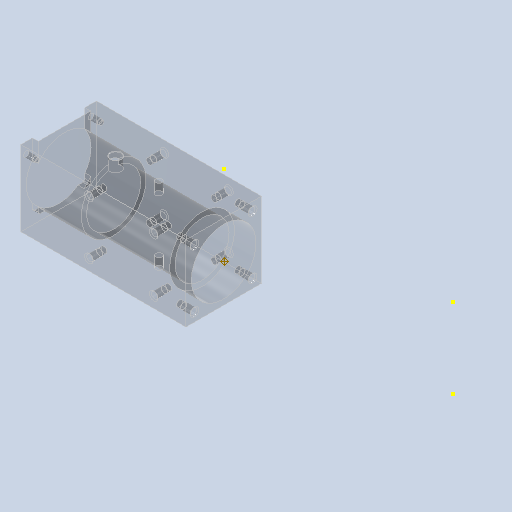
# Autodesk Inventor part: АНЦП.014.00.00.003
Saved by Autodesk Inventor 2022 (Build 260153000, 153)
## iProperties
Created: 2022-02-10
Part Number: АНЦП.014.00.00.003
Material: PET Plastic
Document SubType Name: Modeling
Designer: br4ch
Density: 1.541 g/cm^3
Appearance: Polycarbonate - Clear
Mass: 72.9835 g
Surface Area: 195.713 cm^2
Volume: 47.3611 cm^3
Author: br4ch
Autodesk Inventor part; units mm, degrees
sketch "Sketch1" plane through (0, 0, 0) normal (0, 0, 1) x (1, 0, 0)
  line L0 (-183, -19.5) -> (-106.5, -19.5)
  line L1 (-106.5, -19.5) -> (-106.5, -54.5)
  line L2 (-106.5, -54.5) -> (-183, -54.5)
  line L3 (-183, -54.5) -> (-183, -19.5)
  line L4 (-194, -37) -> (-96, -37) construction
  line L5 (-183, -22) -> (-157.5, -22)
  line L6 (-157.5, -22) -> (-157.5, -37)
  line L7 (-157.5, -24.5) -> (-116.5, -24.5)
  line L8 (-116.5, -37) -> (-116.5, -22)
  line L9 (-116.5, -22) -> (-106.5, -22)
  line L10 (-183, -52) -> (-157.5, -52) construction
  line L11 (-157.5, -52) -> (-157.5, -37) construction
  line L12 (-157.5, -49.5) -> (-116.5, -49.5) construction
  line L13 (-116.5, -37) -> (-116.5, -52) construction
  line L14 (-116.5, -52) -> (-106.5, -52) construction
  line L15 (-183, -37) -> (-106.5, -37)
  point P0 (0, 0)
  dimension "d0" = 76.5
  dimension "d1" = 35
  dimension "d2" = 30
  dimension "d3" = 25.5
  dimension "d4" = 10
  dimension "d5" = 25
  dimension "d6" = 30
  constraints: 32 end point, 9 point on line, 6 symmetric about line, 5 perpendicular, 3 horizontal, 2 midpoint, 2 parallel
  measures "d0" distance of L1.end L2.end
  measures "d1" distance of L0.end L1.end
  measures "d2" distance between parallel lines of L10 L5
  measures "d3" distance of L10.start L10.end
  measures "d4" distance of L13.end L14.end
  measures "d5" distance between parallel lines of L12 L7
  measures "d6" distance between parallel lines of L14 L9
sketch "Sketch3" plane through (0, 0, 0) normal (1, 0, 0) x (0, 1, 0)
  point P0 (0, 0)
ref_plane "Work Plane1" through (-106.5, -37, 0) normal (1, 0, 0) x (0, 1, 0)
sketch "Sketch4" plane through (-106.5, -37, 0) normal (1, 0, 0) x (0, 1, 0)
  point P0 (37, 0)
sketch "Sketch5" plane through (-106.5, -37, 0) normal (1, 0, 0) x (0, 1, 0)
  line L0 (-17.5, 17.5) -> (17.5, 17.5)
  line L1 (17.5, 17.5) -> (17.5, -17.5)
  line L2 (17.5, -17.5) -> (-17.5, -17.5)
  line L3 (-17.5, -17.5) -> (-17.5, 17.5)
  line L4 (-17.5, 17.5) -> (17.5, -17.5) construction
  line L5 (17.5, 17.5) -> (-17.5, -17.5) construction
  point P0 (37, 0)
  point P1 (0, 0)
  dimension "d10" = 35
  dimension "d11" = 35
  constraints: 12 end point, 2 midpoint, 2 parallel, 1 horizontal, 1 perpendicular
  measures "d10" distance of L1.end L2.end
  measures "d11" distance of L0.end L1.end
ref_plane "Work Plane2" through (-183, -37, 0) normal (1, 0, 0) x (0, 1, 0)
extrude "Extrusion1" add sketch "Sketch5" against normal up to surface (76.5 mm away)
revolve "Revolution2" cut sketch "Sketch1" angle 360 about axis through (-194, -37, 0) along (1, 0, 0) contours L5 L6 L15 L3 | L1 L15 L8 L9 | L6 L7 L8 L15
sketch "Sketch7" plane through (-106.5, -37, 0) normal (1, 0, 0) x (0, 0, -1)
  circle A0 centre (0, 0) radius 19.09
  line L0 (-17.5, -17.5) -> (17.5, -17.5) projected
  line L1 (-17.5, 17.5) -> (-17.5, -17.5) projected
  line L2 (17.5, -17.5) -> (-17.5, 17.5) construction
  circle A1 centre (13.4987, -13.4987) radius 1.5
  circle A2 centre (13.4987, 13.4987) radius 1.5
  circle A3 centre (-13.4987, 13.4987) radius 1.5
  circle A4 centre (-13.4987, -13.4987) radius 1.5
  point P0 (0, 37)
  dimension "d21" = 38.18
  dimension "d22" = 3
  dimension "d25" = 360
  constraints: 4 centre point, 2 end point, 1 point on line, 12 other
  measures "d22" diameter of A1
hole "Hole1" at (-106.5, -23.5013, -13.4987) at (-106.5, -23.5013, 13.4987) at (-106.5, -50.4987, 13.4987) at (-106.5, -50.4987, -13.4987) direction (-1, 0, 0) diameter 2.8 depth 7 tip angle 118 counterbore diameter 3 counterbore depth 5
sketch "Sketch8" plane through (-183, -54.5, -17.5) normal (-1, 0, 0) x (0, 0, 1)
  line L0 (17.5, -7) -> (17.5, 46)
  circle A0 centre (2.5, 30) radius 1.25
  line L1 (0, 35) -> (0, 0) projected
  line L2 (35, 35) -> (0, 35) projected
  circle A1 centre (32.5, 30) radius 1.25
  circle A2 centre (17.5, 17.5) radius 15 projected
  circle A3 centre (17.5, 17.5) radius 15 projected
  line L3 (5.3, 6.5) -> (5.3, 35)
  line L4 (0, 35) -> (35, 35) projected
  arc A4 (5.3, 6.5) -> (6.3, 5.5) centre (6.3, 6.5) ccw
  line L5 (17.5, 5.5) -> (6.3, 5.5)
  line L6 (29.7, 6.5) -> (29.7, 35)
  arc A5 (28.7, 5.5) -> (29.7, 6.5) centre (28.7, 6.5) ccw
  line L7 (17.5, 5.5) -> (28.7, 5.5)
  point P0 (17.5, 54.5)
  point P1 (17.5, 5.5)
  point P2 (5.3, 35)
  dimension "d34" = 2.5
  dimension "d35" = 2.5
  dimension "d36" = 5
  dimension "d38" = 1
  dimension "d39" = 29.5
  dimension "d40" = 24.4
  constraints: 10 end point, 6 symmetric about line, 4 centre point, 4 point on circle, 3 perpendicular, 3 point on line, 2 tangent, 1 vertical, 2 other
  measures "d34" diameter of A0
  measures "d35" distance from line of L1 A0.centre
  measures "d36" distance from line of L2 A0.centre
  measures "d38" radius of A4
  measures "d39" distance between parallel lines of L2 L5
  measures "d40" distance between parallel lines of L6 L3
extrude "Extrusion2" cut sketch "Sketch8" against normal blind 2.75 contours L5 A2 L3 L0 | L0 A2 L6 L7 | L5 A4 L3 A2 | A2 L6 A5 L7 | A2 L3 L2 L0 | L0 L2 L6 A2
hole "Hole2" at (-183, -24.5, -15) at (-183, -24.5, 15) direction (1, 0, 0) diameter 2 depth 5 tip angle 118 counterbore diameter 2.5 counterbore depth 4
ref_plane "Work Plane3" through (-106.5, -37, -17.5) normal (0, -1, 0) x (1, 0, 0)
sketch "Sketch9" plane through (-106.5, -37, -17.5) normal (0, -1, 0) x (1, 0, 0)
  point P0 (106.5, 17.5)
sketch "Sketch11" plane through (-106.5, -19.5, 17.5) normal (0, 1, 0) x (1, 0, 0)
  line L0 (-73.75, 5.3) -> (-76.5, 5.3) projected
  line L1 (-76.5, 0) -> (-76.5, 5.3) projected
  line L2 (0, 0) -> (-76.5, 0) projected
  line L3 (0, 35) -> (0, 0) projected
  line L4 (0, 35) -> (-76.5, 35) projected
  line L5 (-76.5, 29.7) -> (-76.5, 35) projected
  line L6 (-76.5, 29.7) -> (-73.75, 29.7) projected
  line L7 (-73.75, 29.7) -> (-73.75, 5.3) projected
  line L8 (28.2317, 17.5) -> (-103.7683, 17.5) construction
  circle A0 centre (-30, 17.5) radius 1.5
  circle A1 centre (-50, 17.5) radius 2.5
  point P0 (106.5, 17.5)
  point P1 (0, 17.5)
  dimension "d54" = 3
  dimension "d55" = 5
  dimension "d56" = 30
  dimension "d57" = 50
  constraints: 3 point on line, 2 centre point, 2 end point, 1 horizontal, 1 midpoint
  measures "d54" diameter of A0
  measures "d55" diameter of A1
  measures "d56" distance from line of A0.centre L3
  measures "d57" distance from line of A1.centre L3
extrude "Extrusion3" cut sketch "Sketch11" against normal up to surface (35 mm away) contours A0
extrude "Extrusion4" cut sketch "Sketch11" against normal up to surface contours A1
sketch "Sketch12" plane through (-106.5, -54.5, -17.5) normal (0, 0, -1) x (-1, 0, 0)
  line L0 (76.5, 35) -> (76.5, 0) projected
  line L1 (0, 35) -> (76.5, 35) projected
  line L2 (0, 0) -> (0, 35) projected
  line L3 (0, 0) -> (76.5, 0) projected
  line L4 (-16, 17.5) -> (90, 17.5)
  circle A0 centre (15, 5) radius 1.5
  circle A1 centre (45, 5) radius 1.5
  circle A2 centre (15, 30) radius 1.5
  circle A3 centre (45, 30) radius 1.5
  point P0 (-106.5, 54.5)
  point P1 (0, 17.5)
  dimension "d62" = 3
  dimension "d63" = 15
  dimension "d64" = 5
  dimension "d67" = 30
  constraints: 4 centre point, 2 end point, 2 horizontal, 2 symmetric about line, 1 midpoint, 1 point on line, 4 other
  measures "d62" diameter of A0
  measures "d63" distance from line of A0.centre L2
  measures "d64" distance from line of L3 A0.centre
  measures "d67" distance of A0.centre A1.centre
hole "Hole3" at (-121.5, -24.5, -17.5) at (-151.5, -24.5, -17.5) at (-151.5, -49.5, -17.5) at (-121.5, -49.5, -17.5) direction (0, 0, 1) diameter 2.8 depth 7 tip angle 118 counterbore diameter 3 counterbore depth 5
ref_plane "Work Plane4" through (-106.5, -54.5, 0) normal (0, 0, -1) x (-1, 0, 0)
mirror "Mirror2" about plane through (-106.5, -54.5, 0) normal (0, 0, -1) of "Hole3"
chamfer "Chamfer3" distance 0.5 angle 45 4 edges at (-151.5, -51, -17.5) (-151.5, -26, -17.5) (-121.5, -51, -17.5) (-121.5, -26, -17.5) measured on face at (-172.9115, -40.8826, -17.5)
chamfer "Chamfer4" distance 0.5 angle 45 4 edges at (-151.5, -26, 17.5) (-151.5, -51, 17.5) (-121.5, -26, 17.5) (-121.5, -51, 17.5) measured on face at (-172.9115, -33.1174, 17.5)
chamfer "Chamfer5" distance 0.5 angle 45 4 edges at (-106.5, -50.4987, -11.9987) (-106.5, -23.5013, -11.9987) (-106.5, -50.4987, 14.9987) (-106.5, -23.5013, 14.9987) measured on face at (-106.5, -37.6027, 16.6302)
chamfer "Chamfer6" distance 0.2 angle 45 1 edges at (-159, -19.5, 0) measured on face at (-148.5662, -19.5, -12.4939)
equation "\"d27\" = m3"
equation "\"d72\" = m3"
equation "\"m3\" = 2.8"
equation "\"m4\" = 3.8"
body "Solid2"
